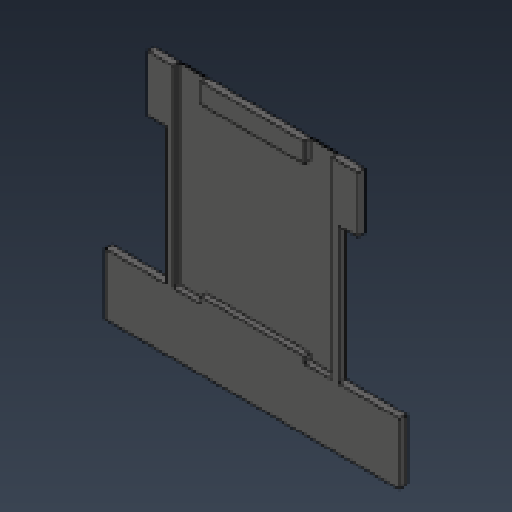
# Autodesk Inventor part: Ceiling
Saved by Autodesk Inventor 2026.2 (Build 302298010, 298A)
## iProperties
Created: 2026-04-07
Part Number: Ceiling
Material: Generic
Document SubType Name: Modeling
Designer: szymo
Density: 1 g/cm^3
Appearance: Default(1)
Author: szymo
Autodesk Inventor part; units mm, degrees
ref_plane "YZ Plane" through (0, 0, 0) normal (1, 0, 0) x (0, 1, 0)
ref_plane "XZ Plane" through (0, 0, 0) normal (0, 1, 0) x (-1, 0, 0)
ref_plane "XY Plane" through (0, 0, 0) normal (0, 0, 1) x (1, 0, 0)
sketch "Sketch1" plane through (0, 0, 0) normal (0, 0, 1) x (1, 0, 0)
  line L0 (-14.25, -14.5) -> (13.65, -14.5)
  line L1 (-13.65, -55.2958) -> (14.25, -55.2958)
  line L2 (50, 0) -> (-50, 0)
  line L3 (-50, 0) -> (-50, -90)
  line L4 (-50, -90) -> (50, -90)
  line L5 (50, -90) -> (50, 0)
  line L6 (-26.85, -65.2958) -> (-26.85, -13) projected
  line L7 (-26.85, -65.2958) -> (-29.35, -65.2958) projected
  line L8 (-29.35, -65.2958) -> (-29.35, -19) projected
  line L9 (-29.35, -19) -> (-35.65, -19) projected
  line L10 (-35.65, -13) -> (-35.65, -19) projected
  line L11 (-26.85, -13) -> (-35.65, -13) projected
  line L12 (26.85, -13) -> (26.85, -65.2958) projected
  line L13 (26.85, -13) -> (35.75, -13) projected
  line L14 (35.75, -19) -> (35.75, -13) projected
  line L15 (29.35, -19) -> (35.75, -19) projected
  line L16 (29.35, -19) -> (29.35, -65.2958) projected
  line L17 (29.35, -65.2958) -> (26.85, -65.2958) projected
  line L18 (-26.85, -3) -> (-26.85, 0) projected
  line L19 (-26.85, -3) -> (-35.65, -3) projected
  line L20 (-35.65, 0) -> (-35.65, -3) projected
  line L21 (-26.85, 0) -> (-35.65, 0) projected
  line L22 (35.75, 0) -> (35.75, -19)
  line L23 (50, -86.2958) -> (-50, -86.2958)
  line L24 (-35.65, 0) -> (-35.65, -19)
  line L25 (14.65, -6.65) -> (-15.25, -6.65)
  line L26 (-15.25, -6.65) -> (-15.25, -22.35)
  line L27 (-15.25, -22.35) -> (14.65, -22.35)
  line L28 (14.65, -22.35) -> (14.65, -6.65)
  line L29 (15.25, -47.4458) -> (-14.65, -47.4458)
  line L30 (-14.65, -47.4458) -> (-14.65, -63.1458)
  line L31 (-14.65, -63.1458) -> (15.25, -63.1458)
  line L32 (15.25, -63.1458) -> (15.25, -47.4458)
  line L33 (30.5, -65.2958) -> (29.35, -65.2958)
  line L34 (-30.5, -65.2958) -> (-29.35, -65.2958)
  circle A0 centre (20.65, -24.0677) radius 2.25 projected
  circle A1 centre (22.6692, -56.1259) radius 2.25 projected
  circle A2 centre (22.25, -13.4966) radius 2.25 projected
  line L35 (19.75, -61.0677) -> (19.75, -50.9236) projected
  line L36 (19.75, -50.9236) -> (23.15, -50.9236) projected
  line L37 (23.15, -50.9236) -> (23.15, -46.7261) projected
  line L38 (19.75, -46.7261) -> (23.15, -46.7261) projected
  line L39 (19.75, -46.7261) -> (19.75, -44.8549) projected
  line L40 (19.75, -44.8549) -> (17.65, -44.8549) projected
  line L41 (17.65, 0) -> (17.65, -44.8549) projected
  line L42 (17.65, 0) -> (26.85, 0) projected
  line L43 (26.85, -65.2958) -> (26.85, 0) projected
  line L44 (23.15, -65.2958) -> (26.85, -65.2958) projected
  line L45 (23.15, -65.2958) -> (23.15, -61.0677) projected
  line L46 (19.75, -61.0677) -> (23.15, -61.0677) projected
  circle A3 centre (-24.3428, -2.5072) radius 2.25 projected
  circle A4 centre (-20.65, -57.8419) radius 2.25 projected
  circle A5 centre (-20.65, -44.9257) radius 2.25 projected
  circle A6 centre (-23.3, -12.9282) radius 2.25 projected
  line L47 (-26.85, 0) -> (-17.65, 0) projected
  line L48 (-17.65, -4.0591) -> (-17.65, 0) projected
  line L49 (-19.75, -4.0591) -> (-17.65, -4.0591) projected
  line L50 (-19.75, -4.7124) -> (-19.75, -4.0591) projected
  line L51 (-19.75, -4.7124) -> (-23.15, -4.7124) projected
  line L52 (-23.15, -4.7124) -> (-23.15, -8.7282) projected
  line L53 (-19.75, -8.7282) -> (-23.15, -8.7282) projected
  line L54 (-19.75, -18.8723) -> (-19.75, -8.7282) projected
  line L55 (-19.75, -18.8723) -> (-23.15, -18.8723) projected
  line L56 (-23.15, -18.8723) -> (-23.15, -23.0697) projected
  line L57 (-19.75, -23.0697) -> (-23.15, -23.0697) projected
  line L58 (-19.75, -24.9409) -> (-19.75, -23.0697) projected
  line L59 (-19.75, -24.9409) -> (-17.65, -24.9409) projected
  line L60 (-17.65, -65.2958) -> (-17.65, -24.9409) projected
  line L61 (-26.85, -65.2958) -> (-17.65, -65.2958) projected
  line L62 (-26.85, 0) -> (-26.85, -65.2958) projected
  line L63 (26.85, 0) -> (26.85, -3) projected
  line L64 (26.85, 0) -> (35.75, 0) projected
  line L65 (35.75, -3) -> (35.75, 0) projected
  line L66 (26.85, -3) -> (35.75, -3) projected
  line L67 (-17.65, -4.0591) -> (-17.65, -24.9409)
  line L68 (23.15, -65.2958) -> (17.65, -65.2958)
  line L69 (17.65, -65.2958) -> (17.65, -44.8549)
  line L70 (17.65, -6.65) -> (-17.65, -6.65)
  line L71 (-17.65, -63.1458) -> (17.65, -63.1458)
  line L72 (34.5, -77.7958) -> (46.525, -77.71) projected
  line L73 (46.525, -77.71) -> (46.525, -78.2976) projected
  arc A7 (46.525, -78.2976) -> (46.9554, -78.442) centre (46.0282, -80.4921) ccw projected
  line L74 (46.9554, -78.442) -> (49, -78.442) projected
  line L75 (49, -78.442) -> (49, -69.922) projected
  line L76 (49, -69.922) -> (46.525, -69.922) projected
  line L77 (46.525, -69.922) -> (34.5, -69.2958) projected
  line L78 (34.5, -69.2958) -> (26.85, -69.2958) projected
  line L79 (26.85, -65.2958) -> (26.85, -69.2958) projected
  line L80 (26.85, -65.2958) -> (50, -65.2958) projected
  line L81 (50, -65.2958) -> (50, -86.2958) projected
  line L82 (34.5, -86.2958) -> (50, -86.2958) projected
  line L83 (34.5, -77.7958) -> (34.5, -86.2958) projected
  arc A8 (-46.9554, -78.442) -> (-46.525, -78.2976) centre (-46.0282, -80.4921) ccw projected
  line L84 (-46.525, -78.2976) -> (-46.525, -77.71) projected
  line L85 (-46.525, -77.71) -> (-34.5, -77.7958) projected
  line L86 (-34.5, -77.7958) -> (-34.5, -86.2958) projected
  line L87 (-34.5, -86.2958) -> (-50, -86.2958) projected
  line L88 (-50, -65.2958) -> (-50, -86.2958) projected
  line L89 (-26.85, -65.2958) -> (-50, -65.2958) projected
  line L90 (-26.85, -65.2958) -> (-26.85, -69.2958) projected
  line L91 (-34.5, -69.2958) -> (-26.85, -69.2958) projected
  line L92 (-34.5, -69.2958) -> (-46.525, -69.922) projected
  line L93 (-46.525, -69.922) -> (-49, -69.922) projected
  line L94 (-49, -69.922) -> (-49, -78.442) projected
  line L95 (-49, -78.442) -> (-46.9554, -78.442) projected
  point P0 (0, 0)
  point P1 (26.95, 0)
  point P2 (26.85, -32.4233)
  point P3 (-15.25, -6.65)
  point P4 (26.85, -13)
  dimension "d0" = 50
  dimension "d1" = 50
  dimension "d2" = 90
  dimension "d3" = 7.85
  dimension "d4" = 7.85
  dimension "d5" = 1
  dimension "d6" = 1
  dimension "d7" = 7.85
  dimension "d8" = 7.85
  dimension "d9" = 1
  dimension "d10" = 1
  dimension "d21" = 0
  constraints: 46 end point, 8 horizontal, 6 perpendicular, 5 parallel, 5 point on line, 3 vertical, 1 collinear, 8 other
  measures "d0" distance from line of L5 point (0, 0)
  measures "d1" distance from line of L3 point (0, 0)
  measures "d2" distance of the line from the sketch origin of L4
  measures "d3" distance between parallel lines of L29 L1
  measures "d4" distance between parallel lines of L31 L1
  measures "d5" distance from line of L32 L1.end
  measures "d6" distance from line of L30 L1.start
  measures "d7" distance between parallel lines of L25 L0
  measures "d8" distance between parallel lines of L27 L0
  measures "d9" distance from line of L28 L0.end
  measures "d10" distance from line of L26 L0.start
  measures "d21" distance between parallel lines of L31 L71
extrude "Extrusion1" add sketch "Sketch1" along normal blind 2 contours L22 L66 L43 L2 | L5 L23 L83 L72 L73 A7 L74 L75 L76 L77 L78 L79 L17 L33 L80 | L22 L13 L43 L66 | L5 L4 L3 L23 | L41 L70 L25 L67 L48 L2 | L14 L15 L16 L17 L12 L13 | L23 L86 L85 L84 A8 L95 L94 L93 L92 L91 L90 L61 L60 L71 L31 L69 L68 L44 L79 L78 L77 L76 L75 L74 A7 L73 L72 L83 | L23 L3 L89 L34 L7 L90 L91 L92 L93 L94 L95 A8 L84 L85 L86 | L18 L19 L20 L2 | L62 L11 L24 L19 | L6 L7 L8 L9 L10 L11
extrude "Extrusion2" add sketch "Sketch1" against normal blind 0.4 contours L22 L66 L43 L2 | L5 L23 L83 L72 L73 A7 L74 L75 L76 L77 L78 L79 L17 L33 L80 | L43 L12 L44 L45 L46 L35 L36 L37 L38 L39 L40 L41 L2 | L22 L13 L43 L66 | L5 L4 L3 L23 | L41 L70 L25 L67 L48 L2 | L14 L15 L16 L17 L12 L13 | L23 L86 L85 L84 A8 L95 L94 L93 L92 L91 L90 L61 L60 L71 L31 L69 L68 L44 L79 L78 L77 L76 L75 L74 A7 L73 L72 L83 | L48 L49 L50 L51 L52 L53 L54 L55 L56 L57 L58 L59 L60 L61 L6 L62 L18 L2 | L41 L69 L71 L32 L29 L30 L60 L67 L70 L26 L27 L28 | L23 L3 L89 L34 L7 L90 L91 L92 L93 L94 L95 A8 L84 L85 L86 | L18 L19 L20 L2 | L67 L59 L58 L57 L56 L55 L54 L53 L52 L51 L50 L49 | L40 L39 L38 L37 L36 L35 L46 L45 L68 L69 | L28 L27 L26 L25 | L62 L11 L24 L19 | L6 L7 L8 L9 L10 L11 | L31 L30 L29 L32 | A0 | A1 | A2 | A3 | A4 | A5 | A6
sketch "Sketch2" plane through (50, -86.2958, 2) normal (1, 0, 0) x (0, 0, -1)
  line L0 (2.2133, 0.4205) -> (-23.8, -4.5217) projected
  line L1 (-23.8, -4.5217) -> (-23.6133, -5.5042) projected
  line L2 (-23.6133, -5.5042) -> (2.4, -0.5619) projected
  line L3 (2.4, -0.5619) -> (2.2133, 0.4205) projected
  line L4 (0, -10.5619) -> (0, 0.2036)
  line L5 (0, 0.2036) -> (2.4, 0.6596)
  line L6 (2.4, 0.6596) -> (2.4, -10.5619)
  line L7 (2.4, -10.5619) -> (0, -10.5619)
  point P0 (2, 86.2958)
  dimension "d15" = 2.4
  dimension "d16" = 0.2
  dimension "d17" = 0
  dimension "d18" = 10
  constraints: 8 end point, 2 vertical, 1 parallel, 1 perpendicular
  measures "d15" distance from line of L4 L2.end
  measures "d16" distance between parallel lines of L5 L0
  measures "d17" distance from line of L6 L2.end
  measures "d18" distance from line of L7 L2.end
extrude "Extrusion3" cut sketch "Sketch2" against normal through all contours L3 L2 L4 L0 | L0 L4 L5 L6 L3 | L6 L7 L4 L2
equation "\"d4\" = d3"
equation "\"d6\" = d5"
equation "\"d7\" = d3"
equation "\"d8\" = d3"
equation "\"d9\" = d5"
equation "\"d10\" = d5"
body "Solid1"
